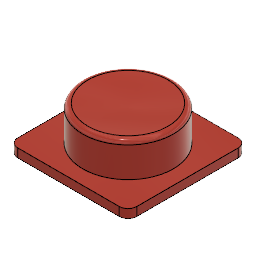
button_ab (Autodesk Fusion 360 design; units mm, degrees)
Autodesk Fusion 360 part; units mm, degrees
sketch "Sketch3" plane through (0, 0, 0) normal (1, 0, 0) x (0, 0, -1)
  line L0 (0, 0) -> (-5.125, 0)
  line L1 (-5.125, 0) -> (-5.125, 4)
  line L2 (0, 0) -> (0, 3.5)
  arc A0 (-5.125, 4) -> (0, 3.5) centre (0.4108, 34.2259) ccw
  dimension "d9" = 5.125
  dimension "d10" = 4
  measures "d9" distance of L0.start L0.end
  measures "d10" distance of L0.end L1.end
revolve "Revolve1" add sketch "Sketch3" angle 360 about axis through (0, 0, 0) along (0, 1, 0)
sketch "Sketch4" plane through (0, 0, 0) normal (0, -1, 0) x (1, 0, 0)
  circle A0 centre (0, 0) radius 5.125
  line L0 (6.75, -6.75) -> (-6.75, -6.75)
  line L1 (-6.75, -6.75) -> (-6.75, 6.75)
  line L2 (-6.75, 6.75) -> (6.75, 6.75)
  line L3 (6.75, 6.75) -> (6.75, -6.75)
  line L4 (6.75, -6.75) -> (-6.75, 6.75) construction
  line L5 (-6.75, -6.75) -> (6.75, 6.75) construction
  dimension "d12" = 13.5
  dimension "d13" = 13.5
  measures "d12" distance of L1.end L2.end
  measures "d13" distance of L0.end L1.end
extrude "Extrude3" add sketch "Sketch4" along normal blind 1 contours A0 | L0 L1 L2 L3
fillet "Fillet2" radius 1 4 edges at (6.75, -0.5, -6.75) (6.75, -0.5, 6.75) (-6.75, -0.5, 6.75) (-6.75, -0.5, -6.75)
fillet "Fillet3" radius 0.5 1 edges at (-4.7782, 4, 1.8533)
sketch "Sketch5" plane through (0, -1, 0) normal (0, -1, 0) x (1, 0, 0)
  arc A0 (-6.75, -5.75) -> (-5.75, -6.75) centre (-5.75, -5.75) ccw
  line L0 (-5.75, -6.75) -> (5.75, -6.75)
  arc A1 (5.75, -6.75) -> (6.75, -5.75) centre (5.75, -5.75) ccw
  line L1 (6.75, -5.75) -> (6.75, 5.75)
  arc A2 (6.75, 5.75) -> (5.75, 6.75) centre (5.75, 5.75) ccw
  line L2 (5.75, 6.75) -> (-5.75, 6.75)
  arc A3 (-5.75, 6.75) -> (-6.75, 5.75) centre (-5.75, 5.75) ccw
  line L3 (-6.75, 5.75) -> (-6.75, -5.75)
  line L4 (1.6, -1.6) -> (-1.6, -1.6)
  line L5 (-1.6, -1.6) -> (-1.6, 1.6)
  line L6 (-1.6, 1.6) -> (1.6, 1.6)
  line L7 (1.6, 1.6) -> (1.6, -1.6)
  line L8 (1.6, -1.6) -> (-1.6, 1.6) construction
  line L9 (-1.6, -1.6) -> (1.6, 1.6) construction
  dimension "d18" = 3.2
  dimension "d19" = 3.2
  measures "d18" distance of L5.end L6.end
  measures "d19" distance of L4.end L5.end
extrude "Extrude4" cut sketch "Sketch5" against normal blind 2.5 contours L4 L5 L6 L7
chamfer "Chamfer1" distance 0.5 angle 45 4 edges at (0, -1, 1.6) (1.6, -1, 0) (0, -1, -1.6) (-1.6, -1, 0)
equation "d9 = ( 10.25 / 2 ) * 1 mm"
